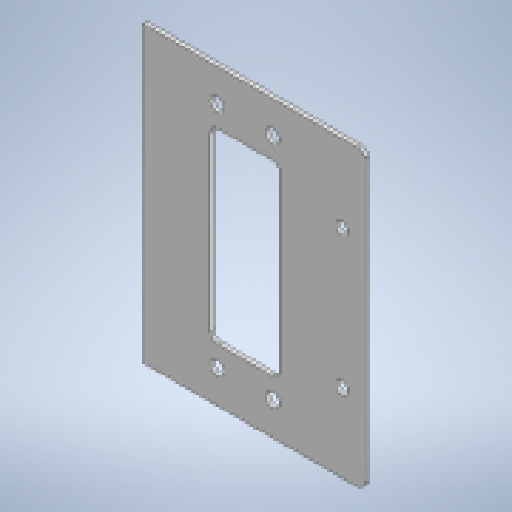
# Autodesk Inventor part: DMF 2.1 01 42 Gear way 2
Saved by Autodesk Inventor 2025 (Build 290162010, 162A)
## iProperties
Created: 2024-04-30
Part Number: DMF 2.1 01 42 Gear way 2
Material: Generic
Document SubType Name: Sheet Metal
Designer: admin
Stock Number: Барабан_Сектор_Усилителя
Density: 1 g/cm^3
Sheet Metal Rule: Default
Sheet Metal Width: 0,000 mm
Sheet Metal Length: 0,000 mm
Sheet Metal Area: 0,000 mm^2
Appearance: Default
Author: pokla
Autodesk Inventor part; units mm, degrees
ref_plane "YZ Plane" through (0, 0, 0) normal (1, 0, 0) x (0, 1, 0)
ref_plane "XZ Plane" through (0, 0, 0) normal (0, 1, 0) x (-1, 0, 0)
ref_plane "XY Plane" through (0, 0, 0) normal (0, 0, 1) x (1, 0, 0)
sketch "Sketch1" plane through (0, 0, 0) normal (0, 0, 1) x (1, 0, 0)
  line L0 (-86.5, 212.492) -> (86.5, 212.492)
  line L1 (86.5, 212.492) -> (86.5, 0)
  line L2 (86.5, 0) -> (-86.5, 0)
  line L3 (-86.5, 0) -> (-86.5, 212.492)
  point P0 (0, 0)
  point P1 (0, 0)
  point P2 (0, 0)
  point P3 (0, 0)
  point P4 (0, 0)
  dimension "d27" = 173
  dimension "d29" = 212.492
  measures "d27" distance of L1.end L2.end
  measures "d29" distance between parallel lines of L2 L0
extrude "Plate1" add sketch "Sketch1" along normal mid plane 3
sketch "Sketch2" plane through (0, 0, 1.5) normal (0, 0, 1) x (1, 0, 0)
  line L0 (-25, 173.746) -> (25, 173.746)
  line L1 (25, 173.746) -> (25, 38.746)
  line L2 (25, 38.746) -> (-25, 38.746)
  line L3 (-25, 38.746) -> (-25, 173.746)
  line L4 (86.5, 212.492) -> (86.5, 0) projected
  line L5 (86.5, 0) -> (-86.5, 0) projected
  circle A0 centre (-20, 188.746) radius 5
  circle A1 centre (20, 188.746) radius 5
  line L6 (-25, 106.246) -> (25, 106.246) construction
  circle A2 centre (-20, 23.746) radius 5
  circle A3 centre (20, 23.746) radius 5
  circle A4 centre (70, 156.246) radius 4.5
  circle A5 centre (70, 56.246) radius 4.5
  line L7 (70, 156.246) -> (70, 56.246) construction
  point P0 (0, 0)
  point P1 (86.5, 106.246)
  point P2 (0, 173.746)
  point P3 (0, 0)
  point P4 (70, 106.246)
  dimension "d33" = 50
  dimension "d34" = 135
  dimension "d35" = 15
  dimension "d36" = 10
  dimension "d37" = 5
  dimension "d38" = 10
  dimension "d39" = 5
  dimension "d43" = 45
  dimension "d44" = 9
  dimension "d45" = 9
  dimension "d46" = 100
  constraints: 12 end point, 6 centre point, 6 midpoint, 3 horizontal alignment, 2 parallel, 2 perpendicular, 2 symmetric about line, 2 vertical alignment, 1 horizontal, 1 vertical, 2 other
  measures "d33" distance of L0.start L0.end
  measures "d34" distance of L0.end L1.end
  measures "d35" vertical distance of L0.start A0.centre
  measures "d36" diameter of A0
  measures "d37" horizontal distance of L0.start A0.centre
  measures "d38" diameter of A1
  measures "d39" horizontal distance of L0.end A1.centre
  measures "d43" horizontal distance of L0.end L7.start
  measures "d44" diameter of A4
  measures "d45" diameter of A5
  measures "d46" distance of L7.end L7.start
extrude "Extrusion1" cut sketch "Sketch2" against normal through all
fillet "Fillet1" radius 5 4 edges at (25, 173.746, 0) (-25, 173.746, 0) (25, 38.746, 0) (-25, 38.746, 0)
sketch "Sketch3" plane through (0, 0, 1.5) normal (0, 0, 1) x (1, 0, 0)
  circle A0 centre (-20, 188.746) radius 5 projected
  circle A1 centre (-20, 23.746) radius 5 projected
  circle A2 centre (20, 188.746) radius 5 projected
  circle A3 centre (70, 156.246) radius 4.5 projected
  circle A4 centre (20, 23.746) radius 5 projected
  line L0 (25, 168.746) -> (25, 43.746) projected
  arc A5 (20, 38.746) -> (25, 43.746) centre (20, 43.746) ccw projected
  line L1 (20, 38.746) -> (-20, 38.746) projected
  arc A6 (-25, 43.746) -> (-20, 38.746) centre (-20, 43.746) ccw projected
  line L2 (-25, 43.746) -> (-25, 168.746) projected
  arc A7 (-20, 173.746) -> (-25, 168.746) centre (-20, 168.746) ccw projected
  line L3 (-20, 173.746) -> (20, 173.746) projected
  arc A8 (25, 168.746) -> (20, 173.746) centre (20, 168.746) ccw projected
  circle A9 centre (70, 56.246) radius 4.5 projected
  line L4 (86.5, 212.492) -> (86.5, 0) projected
  line L5 (-86.5, 212.492) -> (86.5, 212.492) projected
  line L6 (-86.5, 0) -> (-86.5, 212.492) projected
  line L7 (86.5, 0) -> (-86.5, 0) projected
  line L8 (-73.5, 212.492) -> (-73.5, 0)
  point P0 (0, 0)
  dimension "d47" = 13
  constraints: 2 end point, 2 point on line, 1 perpendicular
  measures "d47" distance between parallel lines of L6 L8
extrude "Extrusion2" cut sketch "Sketch3" against normal through all contours L8 L7 L6 L5
fillet "Fillet2" radius 5 2 edges at (86.5, 212.492, 0) (86.5, 0, 0)
equation "\"d33\" = Барабан_Ширина_окна"
equation "\"d34\" = Барабан_Длина_окна"
equation "\"d36\" = Кассета_Диам_шпильки"
equation "\"d38\" = d36"
equation "\"d39\" = d37"
equation "\"d45\" = d44"
equation "\"d15\" = Thickness"
equation "\"BendRadius\" = Thickness"
equation "\"BendReliefWidth\" = Thickness"
equation "\"BendReliefDepth\" = 0.5 * Thickness"
equation "\"CornerReliefSize\" = 4 * Thickness"
equation "\"MinimumRemnant\" = 2 * Thickness"
equation "\"TransitionRadius\" = BendRadius"
equation "\"JacobiRadiusSize\" = BendRadius"
equation "\"GapSize\" = Thickness"
equation "\"Барабан_Ширина_окна\" = 50"
equation "\"Барабан_Длина_окна\" = 135"
equation "\"Кассета_Диам_шпильки\" = 10"
equation "\"Thickness\" = 3"
body "Solid1"
